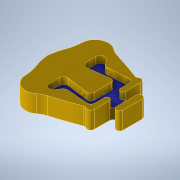
# Autodesk Inventor part: Puma
Saved by Autodesk Inventor 2021 (Build 250183000, 183)
## iProperties
Created: 2020-11-05
Part Number: Puma
Material: Gold
Document SubType Name: Modeling
Designer: IsaacFC
Density: 19.3 g/cm^3
Appearance: Gold
Author: IsaacFC
Autodesk Inventor part; units mm, degrees
ref_plane "YZ Plane" through (0, 0, 0) normal (1, 0, 0) x (0, 1, 0)
ref_plane "XZ Plane" through (0, 0, 0) normal (0, 1, 0) x (-1, 0, 0)
ref_plane "XY Plane" through (0, 0, 0) normal (0, 0, 1) x (1, 0, 0)
sketch "Sketch1" plane through (0, 0, 0) normal (0, 0, 1) x (1, 0, 0)
  line L0 (0, 0) -> (6.3, 0)
  arc A0 (6.3, 0) -> (8.6687, 3.2997) centre (6.3, 2.5) ccw
  line L1 (8.6687, 3.2997) -> (6.6295, 18.4601)
  arc A1 (9.9, 22.2) -> (6.6295, 18.4601) centre (9.9, 18.9) ccw
  line L2 (9.9, 22.2) -> (17.1, 22.2)
  arc A2 (18.9683, 16.1798) -> (17.1, 22.2) centre (17.1, 18.9) ccw
  line L3 (18.9683, 16.1798) -> (15.9184, 14.085)
  arc A3 (15.9184, 14.085) -> (14.4122, 10.9084) centre (17.9, 11.2) ccw
  line L4 (14.4122, 10.9084) -> (15.6913, -4.3917)
  arc A4 (13.2, -7.1) -> (15.6913, -4.3917) centre (13.2, -4.6) ccw
  line L5 (13.2, -7.1) -> (5.9, -7.1)
  arc A5 (5.9, -7.1) -> (5.9, -10.9) centre (5.9, -9) ccw
  line L6 (5.9, -10.9) -> (17.2, -10.9)
  arc A6 (17.2, -10.9) -> (19.1465, -6.8312) centre (17.2, -8.4) ccw
  arc A7 (28.2701, 20.0652) -> (20.7716, 36.0963) centre (20.5, 26.2) ccw
  arc A8 (10.9536, 38.0237) -> (20.7716, 36.0963) centre (21.6, 66.2849) ccw
  arc A9 (10.9536, 38.0237) -> (0, 40.644) centre (-4.9102, -4.0873) ccw
  arc A10 (28.2701, 20.0652) -> (25.6467, 15.0326) centre (40.2, 10.6462) ccw
  arc A11 (18.8493, -4.9649) -> (25.6467, 15.0326) centre (-263.9841, 102.3268) ccw
  arc A12 (18.8493, -4.9649) -> (19.1465, -6.8312) centre (20.6258, -5.6388) ccw
  line L7 (0, 0) -> (0, 50) construction
  line L8 (7.1, -19.6) -> (-7.1, -19.6) construction
  line L9 (7.1, -22) -> (-7.1, -22)
  line L10 (-7.1, -17.2) -> (7.1, -17.2)
  arc A13 (7.1, -22) -> (7.1, -17.2) centre (7.1, -19.6) ccw
  arc A14 (-7.1, -17.2) -> (-7.1, -22) centre (-7.1, -19.6) ccw
  arc A15 (5.9, -10.9) -> (5.9, -17.2) centre (5.9, -14.05) ccw
  line L11 (0, 0) -> (-6.3, 0)
  arc A16 (-8.6687, 3.2997) -> (-6.3, 0) centre (-6.3, 2.5) ccw
  line L12 (-8.6687, 3.2997) -> (-6.6295, 18.4601)
  arc A17 (-6.6295, 18.4601) -> (-9.9, 22.2) centre (-9.9, 18.9) ccw
  line L13 (-9.9, 22.2) -> (-17.1, 22.2)
  arc A18 (-17.1, 22.2) -> (-18.9683, 16.1798) centre (-17.1, 18.9) ccw
  line L14 (-18.9683, 16.1798) -> (-15.9184, 14.085)
  arc A19 (-14.4122, 10.9084) -> (-15.9184, 14.085) centre (-17.9, 11.2) ccw
  line L15 (-14.4122, 10.9084) -> (-15.6913, -4.3917)
  arc A20 (-15.6913, -4.3917) -> (-13.2, -7.1) centre (-13.2, -4.6) ccw
  line L16 (-13.2, -7.1) -> (-5.9, -7.1)
  arc A21 (-5.9, -10.9) -> (-5.9, -7.1) centre (-5.9, -9) ccw
  line L17 (-5.9, -10.9) -> (-17.2, -10.9)
  arc A22 (-19.1465, -6.8312) -> (-17.2, -10.9) centre (-17.2, -8.4) ccw
  arc A23 (-20.7716, 36.0963) -> (-28.2701, 20.0652) centre (-20.5, 26.2) ccw
  arc A24 (-20.7716, 36.0963) -> (-10.9536, 38.0237) centre (-21.6, 66.2849) ccw
  arc A25 (-25.6467, 15.0326) -> (-28.2701, 20.0652) centre (-40.2, 10.6462) ccw
  arc A26 (-25.6467, 15.0326) -> (-18.8493, -4.9649) centre (263.9841, 102.3268) ccw
  arc A27 (-19.1465, -6.8312) -> (-18.8493, -4.9649) centre (-20.6258, -5.6388) ccw
  arc A28 (-5.9, -17.2) -> (-5.9, -10.9) centre (-5.9, -14.05) ccw
  arc A29 (0, 40.644) -> (-10.9536, 38.0237) centre (4.9102, -4.0873) ccw
  point P0 (0, -19.6)
  dimension "d0" = 6.3
  dimension "d1" = 3.3
  dimension "d2" = 3.3
  dimension "d3" = 3.5
  dimension "d4" = 2.5
  dimension "d5" = 1.9
  dimension "d6" = 9.9
  dimension "d7" = 9.9
  dimension "d8" = 18.9
  dimension "d9" = 2.5
  dimension "d10" = 17.1
  dimension "d11" = 11.2
  dimension "d12" = 17.9
  dimension "d13" = 4.6
  dimension "d14" = 13.2
  dimension "d16" = 5.9
  dimension "d18" = 17.2
  dimension "d19" = 8.4
  dimension "d20" = 2.5
  dimension "d21" = 26.2
  dimension "d22" = 1.9
  dimension "d23" = 45
  dimension "d24" = 30.2
  dimension "d25" = 15.2
  dimension "d26" = 302.5
  dimension "d27" = 20.5
  dimension "d28" = 21.6
  dimension "d30" = 40.2
  dimension "d31" = 10.6462
  dimension "d33" = 2.4
  dimension "d34" = 7.1
  dimension "d35" = 19.6
  dimension "d37" = 3.15
  dimension "d38" = 7.1
  constraints: 60 point on circle, 38 end point, 35 symmetric about line, 30 centre point, 23 tangent, 5 horizontal, 2 point on line, 1 midpoint, 1 parallel, 1 vertical, 14 other
  measures "d0" distance of L0.start L0.end
  measures "d1" radius of A1
  measures "d2" radius of A2
  measures "d3" radius of A3
  measures "d4" radius of A4
  measures "d5" radius of A5
  measures "d6" radius of A7
  measures "d7" horizontal distance of A1.centre L0.start
  measures "d8" vertical distance of A1.centre L0.start
  measures "d9" distance of A0.centre L0.end
  measures "d10" horizontal distance of A2.centre L0.start
  measures "d11" vertical distance of A3.centre L0.start
  measures "d12" horizontal distance of L0.start A3.centre
  measures "d13" vertical distance of L0.start A4.centre
  measures "d14" horizontal distance of L0.start A4.centre
  measures "d16" horizontal distance of A5.centre L0.start
  measures "d18" horizontal distance of A6.centre L0.start
  measures "d19" vertical distance of A6.centre L0.start
  measures "d20" radius of A6
  measures "d21" vertical distance of A7.centre L0.start
  measures "d22" radius of A12
  measures "d23" radius of A9
  measures "d24" radius of A8
  measures "d25" radius of A10
  measures "d26" radius of A11
  measures "d27" horizontal distance of L0.start A7.centre
  measures "d28" horizontal distance of L0.start A8.centre
  measures "d30" horizontal distance of L0.start A10.centre
  measures "d31" vertical distance of L0.start A10.centre
  measures "d33" radius of A13
  measures "d34" horizontal distance of L0.start L8.start
  measures "d35" vertical distance of L0.start L8.start
  measures "d37" radius of A15
  measures "d38" horizontal distance of L0.start L8.end
extrude "Extrusion1" add sketch "Sketch1" along normal blind 5 contours L11 A16 L12 A17 L13 A18 L14 A19 L15 A20 L16 A21 L17 A22 A27 A26 A25 A23 A24 A29 A9 A8 A7 A10 A11 A12 A6 L6 A5 L5 A4 L4 A3 L3 A2 L2 A1 L1 A0 L0 | L10 A13 L9 A14
extrude "Extrusion2" add sketch "Sketch1" against normal blind 7.7
body "Solid1"
